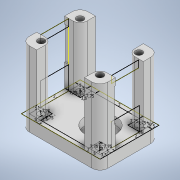
# Autodesk Inventor part: Übersetzungstest_v2
Saved by Autodesk Inventor 2021 (Build 250183000, 183)
## iProperties
Created: 2020-12-31
Part Number: Übersetzungstest_v2
Material: Generisch
Document SubType Name: Modeling
Designer: Ctroi
Density: 1 g/cm^3
Appearance: Vorgabe
Author: Ctroi
## iProperties of the stored document _3D-Druck.ipt
Created: 2020-12-31
Part Number: _3D-Druck
Material: Generisch
Document SubType Name: Modeling
Designer: Ctroi
Density: 1 g/cm^3
Appearance: Vorgabe
Author: Ctroi
Autodesk Inventor part; units mm, degrees
ref_plane "YZ Plane" through (0, 0, 0) normal (1, 0, 0) x (0, 1, 0)
ref_plane "XZ Plane" through (0, 0, 0) normal (0, 1, 0) x (-1, 0, 0)
ref_plane "XY Plane" through (0, 0, 0) normal (0, 0, 1) x (1, 0, 0)
sketch "Skizze1" plane through (0, 0, 0) normal (0, 1, 0) x (-1, 0, 0)
  line L0 (-19.75, -14.75) -> (19.75, -14.75)
  line L1 (19.75, -14.75) -> (19.75, 14.75)
  line L2 (19.75, 14.75) -> (-19.75, 14.75)
  line L3 (-19.75, 14.75) -> (-19.75, -14.75)
  line L4 (0, -20.65) -> (0, 20.65) projected
  line L5 (27.65, 0) -> (-27.65, 0) projected
  point P0 (0, 0)
  dimension "d0" = 39.5
  dimension "d1" = 29.5
  constraints: 8 end point, 2 parallel, 1 horizontal, 1 perpendicular, 2 other
  measures "d0" distance of L1.end L2.end
  measures "d1" distance of L0.end L1.end
extrude "Extrusion1" add sketch "Skizze1" along normal blind 6
sketch "Skizze2" plane through (0, 6, 0) normal (0, 1, 0) x (1, 0, 0)
  line L0 (19.75, 14.75) -> (-19.75, 14.75) projected
  line L1 (-19.75, 14.75) -> (-11.75, 14.75)
  line L2 (-12, 12.75) -> (-12, 7)
  line L3 (-12, 7) -> (-17.75, 7)
  line L4 (-19.75, 6.75) -> (-19.75, 14.75)
  line L5 (19.75, 14.75) -> (10.75, 14.75)
  line L6 (12, 12.75) -> (12, 7)
  line L7 (12, 7) -> (17.75, 7)
  line L8 (19.75, 10.8731) -> (19.75, 14.75)
  line L9 (-19.75, -14.75) -> (19.75, -14.75) projected
  line L10 (-19.75, -14.75) -> (-11.75, -14.75)
  line L11 (-12, -12.75) -> (-12, -7)
  line L12 (-12, -7) -> (-17.75, -7)
  line L13 (-19.75, -6.75) -> (-19.75, -14.75)
  line L14 (19.75, -14.75) -> (11.75, -14.75)
  line L15 (12, -12.75) -> (12, -7)
  line L16 (12, -7) -> (17.75, -7)
  line L17 (19.75, -6.75) -> (19.75, -14.75)
  circle A0 centre (-14.75, 9.75) radius 1.75
  circle A1 centre (-14.75, -9.75) radius 1.75
  circle A2 centre (14.75, -9.75) radius 1.75
  circle A3 centre (14.75, 9.75) radius 1.75
  line L18 (-19.75, 14.75) -> (-19.75, -14.75) projected
  line L19 (-19.75, 14.75) -> (19.75, 14.75)
  line L20 (19.75, 14.75) -> (19.75, -14.75)
  line L21 (19.75, -14.75) -> (-19.75, -14.75)
  line L22 (-19.75, -14.75) -> (-19.75, 14.75)
  line L23 (17.75, 12.75) -> (-17.75, 12.75)
  line L24 (-17.75, 12.75) -> (-17.75, -12.75)
  line L25 (-17.75, -12.75) -> (17.75, -12.75)
  line L26 (17.75, 12.75) -> (17.75, -12.75)
  point P0 (0, 0)
  dimension "d12" = 3.5
  dimension "d13" = 5
  dimension "d14" = 5
  dimension "d15" = 3.5
  dimension "d16" = 5
  dimension "d17" = 5
  dimension "d18" = 3.5
  dimension "d19" = 5
  dimension "d20" = 5
  dimension "d21" = 3.5
  dimension "d22" = 5
  dimension "d23" = 5
  dimension "d24" = 2
  dimension "d25" = 2
  dimension "d28" = 2
  dimension "d29" = 2
  dimension "d30" = 7.75
  dimension "d31" = 7.75
  dimension "d35" = 7.75
  dimension "d36" = 7.75
  dimension "d37" = 7.75
  dimension "d38" = 7.75
  dimension "d39" = 7.75
  dimension "d40" = 7.75
  constraints: 48 end point, 10 parallel, 8 point on line, 6 perpendicular, 5 horizontal, 4 centre point
  measures "d12" diameter of A0
  measures "d13" distance from line of L0 A0.centre
  measures "d14" distance from line of L4 A0.centre
  measures "d15" diameter of A1
  measures "d16" distance from line of L10 A1.centre
  measures "d17" distance from line of L13 A1.centre
  measures "d18" diameter of A2
  measures "d19" distance from line of L17 A2.centre
  measures "d20" distance from line of L14 A2.centre
  measures "d21" diameter of A3
  measures "d22" distance from line of L5 A3.centre
  measures "d23" distance from line of L8 A3.centre
  measures "d24" distance between parallel lines of L0 L23
  measures "d25" distance between parallel lines of L20 L26
  measures "d28" distance between parallel lines of L9 L25
  measures "d29" distance between parallel lines of L22 L24
  measures "d30" distance between parallel lines of L19 L7
  measures "d31" distance between parallel lines of L8 L6
  measures "d35" distance between parallel lines of L4 L2
  measures "d36" distance between parallel lines of L0 L3
  measures "d37" distance between parallel lines of L13 L11
  measures "d38" distance from line of L10.end L12
  measures "d39" distance between parallel lines of L14 L16
  measures "d40" distance between parallel lines of L20 L15
sketch "Skizze3" plane through (0, 6, 0) normal (0, 1, 0) x (1, 0, 0)
  circle A0 centre (5.25, 0) radius 7.7
  line L0 (19.75, -14.75) -> (19.75, 14.75) projected
  line L1 (19.75, 14.75) -> (-19.75, 14.75) projected
  point P0 (0, 0)
  dimension "d32" = 15.4
  dimension "d33" = 14.5
  dimension "d34" = 14.75
  constraints: 1 centre point
  measures "d32" diameter of A0
  measures "d33" distance from line of L0 A0.centre
  measures "d34" distance from line of L1 A0.centre
extrude "Extrusion2" add sketch "Skizze2" along normal blind 31.5 contours L8 L20 L17 L9 L13 L18 L4 L0
extrude "Extrusion3" cut sketch "Skizze3" against normal blind 4
sketch "Skizze4" plane through (5.25, 2, 0) normal (0, 1, 0) x (1, 0, 0)
  circle A0 centre (0, 0) radius 5.3
  point P0 (-5.25, 0)
  dimension "d45" = 10.6
  constraints: 1 centre point
  measures "d45" diameter of A0
extrude "Extrusion4" cut sketch "Skizze4" against normal up to surface (2 mm away)
extrude "Extrusion5" add sketch "Skizze2" along normal blind 31.5 contours L26 L25 L15 L16
extrude "Extrusion6" add sketch "Skizze2" along normal blind 31.5 contours L2 L3 L24 L23 | L23 L26 L7 L6 | L12 L11 L25 L24
extrude "Extrusion7" cut sketch "Skizze2" against normal up to surface (6 mm away) contours A0 | A1 | A2 | A3
fillet "Rundung1" radius 3.5 4 edges at (-12, 21.75, -7) (12, 21.75, -7) (-12, 21.75, 7) (12, 21.75, 7)
fillet "Rundung2" radius 4 4 edges at (19.75, 18.75, 14.75) (19.75, 18.75, -14.75) (-19.75, 18.75, -14.75) (-19.75, 18.75, 14.75)
sketch "Skizze5" plane through (-15.75, 0, 14.75) normal (0, 0, 1) x (1, 0, 0)
  line L0 (3.75, 34) -> (27.75, 34)
  line L1 (27.75, 34) -> (27.75, 17.5)
  line L2 (27.75, 17.5) -> (3.75, 17.5)
  line L3 (3.75, 17.5) -> (3.75, 34)
  line L4 (0, 37.5) -> (31.5, 37.5) projected
  line L5 (-4, 37.5) -> (-4, 0) projected
  line L6 (35.5, 0) -> (35.5, 37.5) projected
  point P0 (15.75, 0)
  dimension "d56" = 16.5
  dimension "d57" = 3.5
  dimension "d58" = 7.75
  dimension "d59" = 7.75
  constraints: 8 end point, 2 parallel, 1 horizontal, 1 perpendicular
  measures "d56" distance of L0.end L1.end
  measures "d57" distance between parallel lines of L4 L0
  measures "d58" distance between parallel lines of L5 L3
  measures "d59" distance between parallel lines of L6 L1
sketch "Skizze6" plane through (15.75, 0, -14.75) normal (0, 0, -1) x (-1, 0, 0)
  line L0 (31.25, 6) -> (27.75, 6) projected
  line L1 (3.75, 34) -> (27.75, 34)
  line L2 (27.75, 34) -> (27.75, 6)
  line L3 (27.75, 6) -> (3.75, 6)
  line L4 (3.75, 6) -> (3.75, 34)
  line L5 (0, 37.5) -> (31.5, 37.5) projected
  point P0 (15.75, 0)
  dimension "d60" = 3.5
  constraints: 8 end point, 2 parallel, 1 horizontal, 1 perpendicular
  measures "d60" distance between parallel lines of L5 L1
extrude "Extrusion8" cut sketch "Skizze6" against normal up to surface (2 mm away)
extrude "Extrusion9" cut sketch "Skizze5" against normal up to surface (2 mm away)
sketch "Skizze7" plane through (-19.75, 0, -10.75) normal (-1, 0, 0) x (0, 0, 1)
  line L0 (3.25, 34) -> (17.25, 34)
  line L1 (17.25, 34) -> (17.25, 17.5)
  line L2 (17.25, 17.5) -> (3.25, 17.5)
  line L3 (3.25, 17.5) -> (3.25, 34)
  line L4 (-4, 37.5) -> (-4, 0) projected
  line L5 (0, 37.5) -> (21.5, 37.5) projected
  point P0 (10.75, 0)
  dimension "d65" = 14
  dimension "d66" = 16.5
  dimension "d67" = 7.25
  dimension "d68" = 3.5
  constraints: 8 end point, 2 parallel, 1 horizontal, 1 perpendicular
  measures "d65" distance of L1.end L2.end
  measures "d66" distance of L0.end L1.end
  measures "d67" distance between parallel lines of L4 L3
  measures "d68" distance between parallel lines of L5 L0
extrude "Extrusion10" cut sketch "Skizze7" against normal up to surface (2 mm away)
sketch "Skizze8" plane through (19.75, 0, 10.75) normal (1, 0, 0) x (0, 0, -1)
  line L0 (3.25, 34) -> (17.25, 34)
  line L1 (17.25, 34) -> (17.25, 17.5)
  line L2 (17.25, 17.5) -> (3.25, 17.5)
  line L3 (3.25, 17.5) -> (3.25, 34)
  line L4 (-4, 37.5) -> (-4, 0) projected
  line L5 (0, 37.5) -> (21.5, 37.5) projected
  point P0 (10.75, 0)
  dimension "d71" = 14
  dimension "d72" = 16.5
  dimension "d73" = 7.25
  dimension "d74" = 3.5
  constraints: 8 end point, 2 parallel, 1 horizontal, 1 perpendicular
  measures "d71" distance of L1.end L2.end
  measures "d72" distance of L0.end L1.end
  measures "d73" distance between parallel lines of L4 L3
  measures "d74" distance between parallel lines of L5 L0
extrude "Extrusion11" cut sketch "Skizze8" against normal up to surface (2 mm away)
sketch "Skizze12" plane through (15.75, 0, -14.75) normal (0, 0, -1) x (-1, 0, 0)
  line L0 (27.75, 34) -> (3.75, 34) projected
  line L1 (27.75, 6) -> (27.75, 37.5) projected
  line L2 (3.75, 34) -> (27.75, 34)
  line L3 (27.75, 34) -> (27.75, 37.5)
  line L4 (27.75, 37.5) -> (3.75, 37.5)
  line L5 (3.75, 37.5) -> (3.75, 34)
  point P0 (15.75, 0)
  constraints: 8 end point, 2 parallel, 1 horizontal, 1 perpendicular
extrude "Extrusion14" cut sketch "Skizze12" against normal up to surface (2 mm away)
sketch "Skizze13" plane through (12, 37.5, 12.75) normal (0, 0, -1) x (-1, 0, 0)
  line L0 (0, 0) -> (0, -31.5) projected
  line L1 (24, -31.5) -> (24, 0) projected
  line L2 (0, -3.5027) -> (24, -3.5027)
  line L3 (24, -3.5027) -> (24, 0)
  line L4 (24, 0) -> (0, 0)
  line L5 (0, 0) -> (0, -3.5027)
  point P0 (12, -37.5)
  point P1 (24, -3.5027)
  constraints: 8 end point, 2 parallel, 1 horizontal, 1 perpendicular, 1 point on line
extrude "Extrusion15" cut sketch "Skizze13" against normal up to surface (2 mm away)
sketch "Skizze14" plane through (-15.75, 0, 14.75) normal (0, 0, 1) x (1, 0, 0)
  line L0 (3.75, 6) -> (3.75, 17.5) projected
  line L1 (27.75, 17.5) -> (27.75, 6) projected
  line L2 (3.75, 17.5) -> (27.75, 17.5)
  line L3 (27.75, 17.5) -> (27.75, 6)
  line L4 (27.75, 6) -> (3.75, 6)
  line L5 (3.75, 6) -> (3.75, 17.5)
  point P0 (15.75, 0)
  point P1 (27.75, 17.5)
  constraints: 8 end point, 2 parallel, 1 horizontal, 1 perpendicular
extrude "Extrusion16" cut sketch "Skizze14" against normal up to surface (2 mm away)
sketch "Skizze15" plane through (-19.75, 0, -10.75) normal (-1, 0, 0) x (0, 0, 1)
  point P0 (10.75, 0)
sketch "Skizze16" plane through (-17.75, 6, 7) normal (1, 0, 0) x (0, 0, -1)
  line L0 (14, 0) -> (0, 0) projected
  line L1 (14, 11.5) -> (14, 28) projected
  line L2 (0, 0) -> (14, 0)
  line L3 (14, 0) -> (14, 11.5)
  line L4 (14, 11.5) -> (0, 11.5)
  line L5 (0, 11.5) -> (0, 0)
  line L6 (0, 31.5) -> (14, 31.5) projected
  line L7 (14, 28) -> (0, 28)
  line L8 (0, 28) -> (0, 31.5)
  line L9 (0, 31.5) -> (14, 31.5)
  line L10 (14, 31.5) -> (14, 28)
  point P0 (7, -6)
  constraints: 16 end point, 4 parallel, 2 horizontal, 2 perpendicular
extrude "Extrusion17" cut sketch "Skizze16" against normal up to surface (2 mm away) contours L6 L10 L7 L8
extrude "Extrusion18" cut sketch "Skizze16" against normal up to surface (2 mm away) contours L0 L5 L4 L3
sketch "Skizze17" plane through (-17.75, 34, 6.5) normal (0, 0, -1) x (-1, 0, 0)
  line L0 (0, 0) -> (2, 0) projected
  line L1 (2, 0) -> (2, -16.5) projected
  line L2 (0, 0) -> (2, 0)
  line L3 (2, 0) -> (2, -16.5)
  line L4 (2, -16.5) -> (0, -16.5)
  line L5 (0, -16.5) -> (0, 0)
  point P0 (-17.75, -34)
  constraints: 8 end point, 2 parallel, 1 horizontal, 1 perpendicular
extrude "Extrusion19" cut sketch "Skizze17" against normal blind 0.5
sketch "Skizze18" plane through (17.75, 6, -7) normal (-1, 0, 0) x (0, 0, 1)
  line L0 (14, 28) -> (14, 31.5) projected
  line L1 (0.5, 28) -> (14, 28) projected
  line L2 (14, 31.5) -> (0.5, 31.5)
  line L3 (0.5, 31.5) -> (0.5, 28)
  line L4 (0.5, 28) -> (14, 28)
  line L5 (14, 28) -> (14, 31.5)
  line L6 (14, 0) -> (0, 0) projected
  line L7 (14.5, 11.5) -> (14, 11.5) projected
  line L8 (0, 0) -> (14, 0)
  line L9 (14, 0) -> (14, 11.5)
  line L10 (14, 11.5) -> (0, 11.5)
  line L11 (0, 11.5) -> (0, 0)
  point P0 (7, -6)
  constraints: 16 end point, 4 parallel, 2 horizontal, 2 perpendicular
extrude "Extrusion20" cut sketch "Skizze18" against normal up to surface (2 mm away) contours L6 L11 L10 L9
extrude "Extrusion21" cut sketch "Skizze18" against normal up to surface (2 mm away) contours L1 L3 L2 L0
sketch "Skizze19" plane through (17.75, 37.5, -6.5) normal (0, 0, 1) x (1, 0, 0)
  line L0 (0, -20) -> (0, 0) projected
  line L1 (2, 0) -> (2, -20) projected
  line L2 (0, -20) -> (2, -20)
  line L3 (2, -20) -> (2, 0)
  line L4 (2, 0) -> (0, 0)
  line L5 (0, 0) -> (0, -20)
  point P0 (-17.75, -37.5)
  constraints: 8 end point, 2 parallel, 1 horizontal, 1 perpendicular
extrude "Extrusion22" cut sketch "Skizze19" against normal blind 0.5
